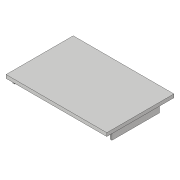
# Autodesk Inventor part: Sharp 2Y0A02 Case Lid
Saved by Autodesk Inventor 2018.3 (Build 223284000, 284)
## iProperties
Created: 2018-12-13
Part Number: Sharp 2Y0A02 Case Lid
Material: Generic
Document SubType Name: Modeling
Designer: aye06091
Mass: 2.51465 g
Surface Area: 36.8923 cm^2
Volume: 2.51465 cm^3
Density: 1 g/cm^3
Appearance: Default
Author: aye06091
Autodesk Inventor part; units mm, degrees
ref_plane "YZ Plane" through (0, 0, 0) normal (1, 0, 0) x (0, 1, 0)
ref_plane "XZ Plane" through (0, 0, 0) normal (0, 1, 0) x (-1, 0, 0)
ref_plane "XY Plane" through (0, 0, 0) normal (0, 0, 1) x (1, 0, 0)
sketch "Sketch1" plane through (0, 0, 0) normal (0, 1, 0) x (-1, 0, 0)
  line L0 (0, 0) -> (-47.9298, 0)
  line L1 (-47.9298, 0) -> (-47.9298, 31.9532)
  line L2 (-47.9298, 31.9532) -> (0, 31.9532)
  line L3 (0, 31.9532) -> (0, 0)
  dimension "d0" = 47.9298
  dimension "d1" = 31.9532
  constraints: 8 end point, 2 parallel, 1 horizontal, 1 perpendicular
  measures "d0" distance of L0.start L0.end
  measures "d1" distance of L2.end L0.start
extrude "Extrusion1" add sketch "Sketch1" along normal blind 1.5875
sketch "Sketch2" plane through (0, 0, 0) normal (0, -1, 0) x (1, 0, 0)
  line L0 (47.9298, 0) -> (47.9298, 31.9532) projected
  line L1 (47.9298, 31.9532) -> (0, 31.9532) projected
  line L2 (0, 31.9532) -> (0, 0) projected
  line L3 (47.5456, 6.4897) -> (46.7265, 6.4897)
  line L4 (46.7265, 6.4897) -> (46.7265, 29.0957)
  line L5 (46.7265, 29.0957) -> (47.5456, 29.0957)
  line L6 (47.5456, 29.0957) -> (47.5456, 6.4897)
  line L7 (1.2033, 29.0957) -> (0.3842, 29.0957)
  line L8 (0.3842, 29.0957) -> (0.3842, 6.4897)
  line L9 (0.3842, 6.4897) -> (1.2033, 6.4897)
  line L10 (1.2033, 6.4897) -> (1.2033, 29.0957)
  line L11 (47.9298, 0) -> (0, 0) projected
  line L12 (0, 0) -> (0, 31.9532) projected
  line L13 (0, 31.9532) -> (47.9298, 31.9532) projected
  line L14 (47.9298, 31.9532) -> (47.9298, 0) projected
  line L15 (0, 0) -> (0, 31.9532) projected
  line L16 (0.3842, 6.4897) -> (1.2033, 6.4897)
  line L17 (1.2033, 6.4897) -> (1.2033, 29.0957)
  line L18 (1.2033, 29.0957) -> (0.3842, 29.0957)
  line L19 (0.3842, 29.0957) -> (0.3842, 6.4897)
  line L20 (47.5456, 29.0957) -> (46.7265, 29.0957)
  line L21 (46.7265, 29.0957) -> (46.7265, 6.4897)
  line L22 (46.7265, 6.4897) -> (47.5456, 6.4897)
  line L23 (47.5456, 6.4897) -> (47.5456, 29.0957)
  dimension "d4" = 22.606
  dimension "d5" = 22.606
  dimension "d6" = 2.8575
  dimension "d7" = 2.8575
  dimension "d8" = 0.3842
  dimension "d9" = 0.3842
  dimension "d10" = 0.8192
  dimension "d11" = 0.8192
  constraints: 32 end point, 8 parallel, 4 horizontal, 4 perpendicular
  measures "d4" distance of L3.end L4.end
  measures "d5" distance of L7.end L8.end
  measures "d6" distance between parallel lines of L1 L5
  measures "d7" distance between parallel lines of L1 L7
  measures "d8" distance between parallel lines of L0 L6
  measures "d9" distance between parallel lines of L2 L8
  measures "d10" distance of L4.end L5.end
  measures "d11" distance between parallel lines of L10 L19
extrude "Extrusion2" add sketch "Sketch2" along normal blind 3.1623 contours L3 L4 L5 L6 | L10 L9 L8 L7
sketch "Sketch3" plane through (0, 0, 0) normal (0, -1, 0) x (1, 0, 0)
  line L0 (47.9298, 31.9532) -> (0, 31.9532) projected
  line L1 (0, 31.9532) -> (0, 0) projected
  line L2 (0.3937, 31.2674) -> (47.5361, 31.2674)
  line L3 (47.5361, 31.2674) -> (47.5361, 30.3657)
  line L4 (47.5361, 30.3657) -> (0.3937, 30.3657)
  line L5 (0.3937, 30.3657) -> (0.3937, 31.2674)
  dimension "d14" = 0.9017
  dimension "d16" = 0.6858
  dimension "d17" = 47.1424
  dimension "d18" = 0.3937
  constraints: 8 end point, 2 parallel, 1 horizontal, 1 perpendicular
  measures "d14" distance between parallel lines of L4 L2
  measures "d16" distance between parallel lines of L0 L2
  measures "d17" distance of L2.start L2.end
  measures "d18" distance between parallel lines of L1 L5
extrude "Extrusion3" cut sketch "Sketch3" against normal blind 0.7937
equation "\"d9\" = d8"
body "Solid1"
